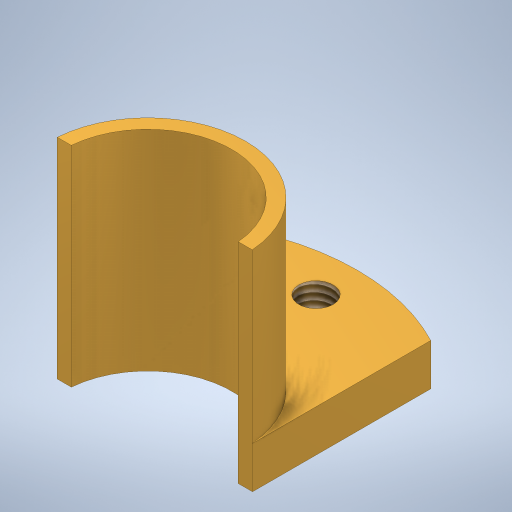
# Autodesk Inventor part: BaffleClamp
Saved by Autodesk Inventor 2024 (Build 280153000, 153)
## iProperties
Created: 2023-10-26
Part Number: BaffleClamp
Material: Brass, Soft Yellow
Document SubType Name: Modeling
Designer: schanen
Density: 8.47 g/cm^3
Appearance: Brass - Satin
Author: schanen
Autodesk Inventor part; units mm, degrees
ref_plane "YZ Plane" through (0, 0, 0) normal (1, 0, 0) x (0, 1, 0)
ref_plane "XZ Plane" through (0, 0, 0) normal (0, 1, 0) x (-1, 0, 0)
ref_plane "XY Plane" through (0, 0, 0) normal (0, 0, 1) x (1, 0, 0)
sketch "Sketch1" plane through (0, 0, 0) normal (0, 0, 1) x (1, 0, 0)
  line L0 (-15, 0) -> (-6, 0)
  line L1 (-6, 0) -> (-6, 15)
  line L2 (-6, 15) -> (-7, 15)
  line L3 (-7, 15) -> (-7, 3)
  line L4 (-7, 3) -> (-15, 3)
  line L5 (-15, 3) -> (-15, 0)
  line L6 (0, -3) -> (0, 18) projected
  point P0 (0, 0)
  dimension "d0" = 3
  dimension "d1" = 1
  dimension "d2" = 15
  dimension "d3" = 6
  dimension "d4" = 15
  constraints: 12 end point, 4 perpendicular, 1 horizontal, 1 horizontal alignment, 1 parallel
  measures "d0" distance of L4.end L0.start
  measures "d1" distance between parallel lines of L1 L3
  measures "d2" distance of L0.end L1.end
  measures "d3" distance from line of point (0, 0) L1
  measures "d4" distance from line of point (0, 0) L5
revolve "Revolution1" add sketch "Sketch1" angle 360 about axis through (0, -10, 0) along (0, 1, 0)
sketch "Sketch2" plane through (0, 3, 0) normal (0, 1, 0) x (1, 0, 0)
  point P0 (0, 0)
  point P1 (0.0472, 12)
  dimension "d6" = 12
  measures "d6" vertical distance of point (0, 0) point (0.047, 12)
hole "Hole1" at (0.0472, 3, -12) direction (0, -1, 0) diameter 2.459 end through all thread size "M3x0.5" class "6H" standard "ISO Metric profile"
sketch "Sketch3" plane through (0, 15, 0) normal (0, 1, 0) x (1, 0, 0)
  line L0 (-15, 0.5) -> (15, 0.5)
  line L1 (15, 0.5) -> (15, -15)
  line L2 (15, -15) -> (-15, -15)
  line L3 (-15, -15) -> (-15, 0.5)
  circle A0 centre (0, 0) radius 15 projected
  line L4 (-15, 0) -> (-7, 0)
  line L5 (-7, 0) -> (-7, 15)
  line L6 (-7, 15) -> (-15, 15)
  line L7 (-15, 15) -> (-15, 0)
  circle A1 centre (0, 0) radius 7 projected
  line L8 (15, 0) -> (7, 0)
  line L9 (7, 0) -> (7, 15)
  line L10 (7, 15) -> (15, 15)
  line L11 (15, 15) -> (15, 0)
  point P0 (14.9917, 0.5)
  point P1 (-14.9917, 0.5)
  point P2 (7, 0.5)
  point P3 (-7, 0.5)
  point P4 (-7, 13.2665)
  dimension "d14" = 0.5
  constraints: 24 end point, 7 tangent, 6 parallel, 3 horizontal, 3 perpendicular, 2 point on circle, 2 point on line
  measures "d14" distance from line of point (0, 0) L0
extrude "Extrusion1" cut sketch "Sketch3" against normal through all contours A0 L5 L0 | L0 L5 L4 A0 | A0 L2 L3 | L4 A1 L8 A0 | L0 A1 L5 | A0 L1 L2 | A1 L0 | L9 L10 L11 L0 A0 | A0 L0 L9 | L8 L9 L0 A0 | A1 L0 L9 picked at (0.8274, -1.8484)
body "Solid1"
